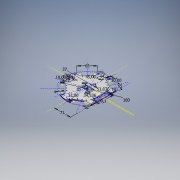
# Autodesk Inventor part: lower_baseplate_collet_alu
Saved by Autodesk Inventor 2018 (Build 220112000, 112)
## iProperties
Created: 2017-08-19
Part Number: lower_baseplate_collet_alu
Material: Aluminum 6061
Document SubType Name: Modeling
Designer: steve
Mass: 141.906 g
Surface Area: 381.464 cm^2
Volume: 52.5578 cm^3
Density: 2.7 g/cm^3
Appearance: Aluminum - Flat
Author: steve
Autodesk Inventor part; units mm, degrees
ref_plane "YZ Plane" through (0, 0, 0) normal (1, 0, 0) x (0, 1, 0)
ref_plane "XZ Plane" through (0, 0, 0) normal (0, 1, 0) x (-1, 0, 0)
ref_plane "XY Plane" through (0, 0, 0) normal (0, 0, 1) x (1, 0, 0)
sketch "Sketch1" plane through (0, 0, 0) normal (0, 0, 1) x (1, 0, 0)
  arc A0 (71, -55.3082) -> (70.1094, -56.433) centre (0, 0) ccw construction
  line L0 (-177.0006, 0) -> (176.9983, 0) construction
  line L1 (0, -176.9989) -> (0, 177.0006) construction
  line L2 (0, 0) -> (-102.7393, 102.7393) construction
  line L3 (0, 0) -> (65.4836, 113.4209) construction
  line L4 (0, 0) -> (-102.7393, -102.7393) construction
  line L5 (0, 0) -> (65.4836, -113.4209) construction
  arc A1 (-63.6396, 63.6396) -> (-82.3264, 36.3644) centre (0, 0) ccw construction
  line L6 (-86.6206, 40.6586) -> (-40.6586, 86.6206) construction
  line L7 (-40.6586, 86.6206) -> (-36.3644, 82.3264) construction
  line L8 (-25.1023, 71.0642) -> (-71.0642, 25.1023)
  line L9 (-71.0642, 25.1023) -> (-82.3264, 36.3644)
  line L10 (-63.6396, 63.6396) -> (-48.0833, 48.0833) construction
  line L11 (5.8542, 75.1397) -> (62.1458, 42.6397)
  line L12 (62.1458, 42.6397) -> (70.1094, 56.433)
  line L13 (73.1458, 61.6923) -> (16.8542, 94.1923) construction
  line L14 (16.8542, 94.1923) -> (13.8177, 88.933) construction
  line L15 (45, 77.9423) -> (34, 58.8897) construction
  line L16 (-36.3644, 82.3264) -> (-25.1023, 71.0642)
  line L17 (-82.3264, 36.3644) -> (-86.6206, 40.6586) construction
  line L18 (13.8177, 88.933) -> (5.8542, 75.1397)
  line L19 (70.1094, 56.433) -> (73.1458, 61.6923) construction
  arc A2 (-36.3644, 82.3264) -> (-63.6396, 63.6396) centre (0, 0) ccw construction
  arc A3 (-82.3264, 36.3644) -> (-90, 0) centre (0, 0) ccw
  arc A4 (13.8177, 88.933) -> (-36.3644, 82.3264) centre (0, 0) ccw
  arc A5 (45, 77.9423) -> (13.8177, 88.933) centre (0, 0) ccw construction
  arc A6 (70.1094, 56.433) -> (45, 77.9423) centre (0, 0) ccw construction
  arc A7 (-90, 0) -> (90, 0) centre (0, 0) ccw construction
  arc A8 (90, 0) -> (71, 55.3082) centre (0, 0) ccw construction
  line L20 (0, 0) -> (-102.7393, -102.7393) construction
  line L21 (0, 0) -> (65.4836, -113.4209) construction
  arc A9 (-82.3264, -36.3644) -> (-63.6396, -63.6396) centre (0, 0) ccw construction
  line L22 (-86.6206, -40.6586) -> (-40.6586, -86.6206) construction
  line L23 (-40.6586, -86.6206) -> (-36.3644, -82.3264) construction
  line L24 (-25.1023, -71.0642) -> (-71.0642, -25.1023)
  line L25 (-71.0642, -25.1023) -> (-82.3264, -36.3644)
  line L26 (-63.6396, -63.6396) -> (-48.0833, -48.0833) construction
  line L27 (5.8542, -75.1397) -> (62.1458, -42.6397)
  line L28 (62.1458, -42.6397) -> (70.1094, -56.433)
  line L29 (73.1458, -61.6923) -> (16.8542, -94.1923) construction
  line L30 (16.8542, -94.1923) -> (13.8177, -88.933) construction
  line L31 (45, -77.9423) -> (34, -58.8897) construction
  line L32 (-36.3644, -82.3264) -> (-25.1023, -71.0642)
  line L33 (-82.3264, -36.3644) -> (-86.6206, -40.6586) construction
  line L34 (13.8177, -88.933) -> (5.8542, -75.1397)
  line L35 (70.1094, -56.433) -> (73.1458, -61.6923) construction
  arc A10 (-63.6396, -63.6396) -> (-36.3644, -82.3264) centre (0, 0) ccw construction
  arc A11 (-90, 0) -> (-82.3264, -36.3644) centre (0, 0) ccw
  arc A12 (-36.3644, -82.3264) -> (13.8177, -88.933) centre (0, 0) ccw
  arc A13 (13.8177, -88.933) -> (45, -77.9423) centre (0, 0) ccw construction
  arc A14 (45, -77.9423) -> (70.1094, -56.433) centre (0, 0) ccw construction
  arc A15 (70.1094, -56.433) -> (71, -55.3082) centre (0, 0) ccw
  line L36 (71, 115.675) -> (71, -111.017) construction
  line L37 (71, -55.3082) -> (71, 55.3082)
  arc A16 (71, 55.3082) -> (70.1094, 56.433) centre (0, 0) ccw
  arc A17 (70.1094, -56.433) -> (71, -55.3082) centre (0, 0) ccw construction
  arc A18 (71, -55.3082) -> (90, 0) centre (0, 0) ccw construction
  dimension "d0" = 180
  dimension "d1" = 45
  dimension "d2" = 30
  dimension "d5" = 22
  dimension "d6" = 65
  dimension "d7" = 22
  dimension "d8" = 65
  dimension "d26" = 71
  constraints: 72 end point, 46 point on circle, 19 centre point, 18 symmetric about line, 9 parallel, 8 perpendicular, 4 midpoint, 4 point on line, 3 coincident, 3 tangent, 2 collinear, 1 vertical, 7 other
  measures "d0" diameter of A0
  measures "d1" angle of L1 L2
  measures "d2" angle of L3 L1
  measures "d5" distance of L6.end L8.start
  measures "d6" distance of L6.start L6.end
  measures "d7" distance of L13.end L11.start
  measures "d8" distance of L13.start L13.end
  measures "d26" distance between parallel lines of L1 L36
extrude "Extrusion1" add sketch "Sketch1" along normal blind 3
sketch "Sketch3" plane through (0, 0, 0) normal (0, 0, -1) x (-1, 0, 0)
  line L0 (0, 0) -> (48.0833, 48.0833) construction
  line L1 (25.1023, 71.0642) -> (71.0642, 25.1023) construction
  line L2 (0, 0) -> (-34, 58.8897) construction
  line L3 (-62.1458, 42.6397) -> (-5.8542, 75.1397) construction
  line L4 (68.9101, 27.2565) -> (27.6205, 68.546) construction
  line L5 (-11.9462, 71.6225) -> (-60.3861, 43.6557) construction
  line L6 (63.8841, 25.9184) -> (21.8996, 67.903) construction
  line L7 (-13.3687, 65.6051) -> (-54.2429, 42.0063) construction
  line L8 (122.2004, 0) -> (-103.2027, 0) construction
  point P0 (44.9013, 44.9013)
  point P1 (-31.75, 54.9926)
  point P2 (54.8008, 35.0018)
  point P3 (-19.6256, 61.9926)
  point P4 (35.0018, 54.8008)
  point P5 (-43.8744, 47.9926)
  point P6 (44.9013, -44.9013)
  point P7 (-31.75, -54.9926)
  point P8 (54.8008, -35.0018)
  point P9 (-19.6256, -61.9926)
  point P10 (35.0018, -54.8008)
  point P11 (-43.8744, -47.9926)
  dimension "d13" = 0
  dimension "d14" = 0
  dimension "d15" = 4.5
  dimension "d16" = 4.5
  dimension "d17" = 14
  dimension "d18" = 14
  constraints: 12 end point, 8 symmetric about line, 6 point on line, 2 midpoint, 2 parallel, 2 perpendicular
  measures "d13" distance between parallel lines of L4 L1
  measures "d14" distance between parallel lines of L5 L3
  measures "d15" distance between parallel lines of L6 L4
  measures "d16" distance between parallel lines of L5 L7
  measures "d17" distance of point (54.801, 35.002) point (44.901, 44.901)
  measures "d18" distance of point (-31.75, 54.993) point (-19.626, 61.993)
hole "Hole1" at (-44.9013, 44.9013, 0) at (31.75, 54.9926, 0) at (-54.8008, 35.0018, 0) at (19.6256, 61.9926, 0) at (-35.0018, 54.8008, 0) at (43.8744, 47.9926, 0) at (-54.8008, -35.0018, 0) at (-44.9013, -44.9013, 0) at (-35.0018, -54.8008, 0) at (19.6256, -61.9926, 0) at (31.75, -54.9926, 0) at (43.8744, -47.9926, 0) direction (0, 0, 1) diameter 3 end through all countersink diameter 6 countersink angle 90
sketch "Sketch5" plane through (0, 0, 3) normal (0, 0, 1) x (1, 0, 0)
  circle A0 centre (31.75, -54.9926) radius 1.5 construction
  circle A1 centre (-35.0018, -54.8008) radius 1.5 construction
  circle A2 centre (-54.8008, -35.0018) radius 1.5 construction
  circle A3 centre (-35.0018, 54.8008) radius 1.5 construction
  circle A4 centre (-54.8008, 35.0018) radius 1.5 construction
  circle A5 centre (-44.9013, 44.9013) radius 1.5 construction
  circle A6 centre (31.75, 54.9926) radius 1.5 construction
  circle A7 centre (19.6256, 61.9926) radius 1.5 construction
  circle A8 centre (43.8744, 47.9926) radius 1.5 construction
  circle A9 centre (-44.9013, -44.9013) radius 1.5 construction
  circle A10 centre (19.6256, -61.9926) radius 1.5 construction
  circle A11 centre (43.8744, -47.9926) radius 1.5 construction
  line L0 (-25.1023, 71.0642) -> (-71.0642, 25.1023) construction
  line L1 (-71.0642, 25.1023) -> (-82.3264, 36.3644) construction
  arc A12 (-82.3264, 36.3644) -> (-82.3264, -36.3644) centre (0, 0) ccw construction
  line L2 (-82.3264, -36.3644) -> (-71.0642, -25.1023) construction
  line L3 (-71.0642, -25.1023) -> (-25.1023, -71.0642) construction
  line L4 (-25.1023, -71.0642) -> (-36.3644, -82.3264) construction
  arc A13 (-36.3644, -82.3264) -> (13.8177, -88.933) centre (0, 0) ccw construction
  line L5 (13.8177, -88.933) -> (5.8542, -75.1397) construction
  line L6 (5.8542, -75.1397) -> (62.1458, -42.6397) construction
  line L7 (62.1458, -42.6397) -> (70.1094, -56.433) construction
  arc A14 (70.1094, -56.433) -> (71, -55.3082) centre (0, 0) ccw construction
  line L8 (71, -55.3082) -> (71, 55.3082) construction
  arc A15 (71, 55.3082) -> (70.1094, 56.433) centre (0, 0) ccw construction
  line L9 (70.1094, 56.433) -> (62.1458, 42.6397) construction
  line L10 (62.1458, 42.6397) -> (5.8542, 75.1397) construction
  line L11 (5.8542, 75.1397) -> (13.8177, 88.933) construction
  arc A16 (13.8177, 88.933) -> (-36.3644, 82.3264) centre (0, 0) ccw construction
  line L12 (-36.3644, 82.3264) -> (-25.1023, 71.0642) construction
  line L13 (71, -55.3082) -> (71, 55.3082) construction
  line L14 (71, -46.5) -> (44, -46.5) construction
  line L15 (44, -46.5) -> (44, 46.5) construction
  line L16 (44, 46.5) -> (71, 46.5) construction
  line L17 (71, 46.5) -> (71, -46.5) construction
  line L18 (71, -31.5) -> (54, -31.5)
  line L19 (54, -31.5) -> (54, 31.5)
  line L20 (54, 31.5) -> (71, 31.5)
  line L21 (71, 31.5) -> (71, -31.5)
  line L22 (-122.2004, 0) -> (103.2027, 0) construction
  line L23 (44, 0) -> (71, 0) construction
  line L24 (54, 0) -> (71, 0) construction
  dimension "d27" = 93
  dimension "d28" = 27
  dimension "d30" = 63
  dimension "d57" = 17
  constraints: 20 end point, 4 midpoint, 4 parallel, 3 perpendicular, 2 collinear, 2 horizontal, 2 point on line
  measures "d27" distance between parallel lines of L16 L14
  measures "d28" distance of L15.end L16.end
  measures "d30" distance of L18.end L19.end
  measures "d57" distance of L18.start L18.end
fillet "Fillet1" radius 10 6 edges at (5.8542, -75.1397, 1.5) (-25.1023, -71.0642, 1.5) (-71.0642, -25.1023, 1.5) (-71.0642, 25.1023, 1.5) (-25.1023, 71.0642, 1.5) (5.8542, 75.1397, 1.5)
ref_plane "Work Plane1" through (0, 0, 3) normal (0, -1, 0) x (1, 0, 0)
extrude "Extrusion3" cut sketch "Sketch5" against normal through all
sketch "Sketch7" plane through (0, 0, 0) normal (0, 0, -1) x (-1, 0, 0)
  line L0 (50.681, 5.7797) -> (-5.2133, -50.1146) construction
  line L1 (63.9932, -32.1734) -> (32.1734, -63.9932) construction
  line L2 (15.0888, -45.3733) -> (-48.6749, -8.5593) construction
  line L3 (-14.5144, -70.1397) -> (-62.1458, -42.6397) construction
  line L4 (33.0572, -11.844) -> (27.4004, -17.5009)
  line L5 (27.4004, -17.5009) -> (25.2791, -15.3796)
  line L6 (25.2791, -15.3796) -> (30.9359, -9.7227)
  line L7 (30.9359, -9.7227) -> (33.0572, -11.844)
  line L8 (0, 0) -> (102.7393, -102.7393) construction
  line L9 (11.844, -33.0572) -> (17.5009, -27.4004)
  line L10 (17.5009, -27.4004) -> (15.3796, -25.2791)
  line L11 (15.3796, -25.2791) -> (9.7227, -30.9359)
  line L12 (9.7227, -30.9359) -> (11.844, -33.0572)
  line L13 (-2.8846, -34.9963) -> (-9.8128, -30.9963)
  line L14 (-9.8128, -30.9963) -> (-8.3878, -28.5281)
  line L15 (-8.3878, -28.5281) -> (-1.4596, -32.5281)
  line L16 (-1.4596, -32.5281) -> (-2.8846, -34.9963)
  line L17 (0, 0) -> (-65.4836, -113.4209) construction
  line L18 (-28.8654, -19.9963) -> (-21.9372, -23.9963)
  line L19 (-21.9372, -23.9963) -> (-20.5122, -21.5281)
  line L20 (-20.5122, -21.5281) -> (-27.4404, -17.5281)
  line L21 (-27.4404, -17.5281) -> (-28.8654, -19.9963)
  line L22 (177.0006, 0) -> (-176.9983, 0) construction
  line L23 (33.0572, 11.844) -> (27.4004, 17.5009)
  line L24 (27.4004, 17.5009) -> (25.2791, 15.3796)
  line L25 (25.2791, 15.3796) -> (30.9359, 9.7227)
  line L26 (30.9359, 9.7227) -> (33.0572, 11.844)
  line L27 (9.7227, 30.9359) -> (11.844, 33.0572)
  line L28 (15.3796, 25.2791) -> (9.7227, 30.9359)
  line L29 (17.5009, 27.4004) -> (15.3796, 25.2791)
  line L30 (11.844, 33.0572) -> (17.5009, 27.4004)
  line L31 (-2.8846, 34.9963) -> (-9.8128, 30.9963)
  line L32 (-9.8128, 30.9963) -> (-8.3878, 28.5281)
  line L33 (-8.3878, 28.5281) -> (-1.4596, 32.5281)
  line L34 (-1.4596, 32.5281) -> (-2.8846, 34.9963)
  line L35 (-27.4404, 17.5281) -> (-28.8654, 19.9963)
  line L36 (-20.5122, 21.5281) -> (-27.4404, 17.5281)
  line L37 (-21.9372, 23.9963) -> (-20.5122, 21.5281)
  line L38 (-28.8654, 19.9963) -> (-21.9372, 23.9963)
  point P0 (-55.5466, -46.4498)
  point P1 (-53.4856, -47.6397)
  dimension "d45" = 36.25
  dimension "d46" = 36.25
  dimension "d47" = 3
  dimension "d48" = 8
  dimension "d49" = 15
  dimension "d51" = 8
  dimension "d52" = 2.85
  dimension "d53" = 15
  constraints: 68 end point, 24 symmetric about line, 4 parallel, 4 perpendicular, 4 point on line
  measures "d45" distance between parallel lines of L0 L1
  measures "d46" distance between parallel lines of L2 L3
  measures "d47" distance of L6.end L4.start
  measures "d48" distance of L5.end L6.end
  measures "d49" distance between parallel lines of L8 L7
  measures "d51" distance of L13.start L13.end
  measures "d52" distance of L15.end L13.start
  measures "d53" distance between parallel lines of L17 L16
extrude "Extrusion2" [suppressed]
fillet "Fillet2" radius 2 10 edges at (13.8177, 88.933, 1.5) (70.1094, 56.433, 1.5) (-82.3264, 36.3644, 1.5) (-36.3644, 82.3264, 1.5) (-82.3264, -36.3644, 1.5) (-36.3644, -82.3264, 1.5) (13.8177, -88.933, 1.5) (70.1094, -56.433, 1.5) (71, -55.3082, 1.5) (71, 55.3082, 1.5)
sketch "Sketch9" plane through (0, 0, 0) normal (0, 0, -1) x (-1, 0, 0)
  line L0 (-54, -31.5) -> (-54, 31.5) construction
  line L1 (-54, 0) -> (-20.2293, 0) construction
  line L2 (-54, -10.05) -> (-19.464, -10.05)
  line L3 (-19.464, -10.05) -> (-19.464, 10.05)
  line L4 (-19.464, 10.05) -> (-54, 10.05)
  line L5 (-54, 10.05) -> (-54, -10.05)
  line L6 (-54, 0) -> (-19.464, 0) construction
  line L7 (-54, 31.5) -> (-54, -31.5) construction
  point P0 (0, 0)
  dimension "d70" = 20.1
  dimension "d71" = 34.536
  constraints: 12 end point, 3 midpoint, 2 collinear, 2 horizontal, 2 parallel, 1 perpendicular
  measures "d70" distance between parallel lines of L2 L4
  measures "d71" distance between parallel lines of L3 L0
sketch "Sketch10" plane through (0, 0, 0) normal (0, 0, -1) x (-1, 0, 0)
  circle A0 centre (0, 0) radius 26 construction
  line L0 (-5.4644, -42.234) -> (43.0476, 6.278) construction
  line L1 (63.9932, -32.1734) -> (32.1734, -63.9932) construction
  line L2 (0, 0) -> (102.7393, -102.7393) construction
  line L3 (20.5061, -20.5061) -> (9.8995, -31.1127) construction
  line L4 (-27.0128, -14.4264) -> (-1.5766, -29.112) construction
  line L5 (-14.5144, -70.1397) -> (-62.1458, -42.6397) construction
  line L6 (-14.5, -25.1147) -> (-27.4904, -17.6147) construction
  line L7 (0, 0) -> (-65.4836, -113.4209) construction
  line L8 (177.0006, 0) -> (-176.9983, 0) construction
  point P0 (18.3848, -18.3848)
  point P1 (31.1127, -9.8995)
  point P2 (-53.4856, -47.6397)
  point P3 (-13, -22.5167)
  point P4 (-1.5096, -32.6147)
  point P5 (9.8995, 31.1127)
  point P6 (18.3848, 18.3848)
  point P7 (31.1127, 9.8995)
  point P8 (-27.4904, 17.6147)
  point P9 (-13, 22.5167)
  point P10 (-1.5096, 32.6147)
  dimension "d72" = 42
  dimension "d75" = 15
  dimension "d76" = 3
  dimension "d77" = 15
  dimension "d78" = 3
  constraints: 8 end point, 8 symmetric about line, 6 point on line, 3 coincident, 2 parallel, 2 perpendicular, 2 tangent, 1 centre point
  measures "d72" distance between parallel lines of L1 L0
  measures "d75" distance of L3.start L3.end
  measures "d76" distance between parallel lines of L0 L3
  measures "d77" distance of L6.start L6.end
  measures "d78" distance between parallel lines of L4 L6
hole "Hole3" [suppressed]
sketch "Sketch11" plane through (0, 0, 0) normal (0, 0, -1) x (-1, 0, 0)
  circle A0 centre (9.0389, -68.6576) radius 17.75 construction
  arc A1 (-10.8406, -89.3447) -> (33.5954, -83.4946) centre (0, 0) ccw construction
  line L0 (11.7474, -89.23) -> (0, 0) construction
  circle A2 centre (9.0389, -68.6576) radius 11 construction
  line L1 (177.0006, 0) -> (-176.9983, 0) construction
  point P0 (11.3558, -86.2557)
  point P1 (10.4747, -79.5635)
  point P2 (17.7658, -61.9612)
  point P3 (-1.1237, -64.448)
  point P4 (10.4747, 79.5635)
  point P5 (17.7658, 61.9612)
  point P6 (-1.1237, 64.448)
  dimension "d86" = 35.5
  dimension "d88" = 22
  dimension "d87" = 3
  dimension "d91" = 360
  constraints: 3 point on line, 3 symmetric about line, 2 end point, 1 coincident, 1 point on circle, 10 other
  measures "d87" distance of L0.start point (11.356, -86.256)
hole "Hole4" at (-10.4747, -79.5635, 0) at (-17.7658, -61.9612, 0) at (1.1237, -64.448, 0) at (-10.4747, 79.5635, 0) at (1.1237, 64.448, 0) at (-17.7658, 61.9612, 0) direction (0, 0, 1) diameter 3 depth 8 tip angle 118 countersink diameter 6 countersink angle 90
sketch "Sketch12" plane through (0, 0, 0) normal (0, 0, -1) x (-1, 0, 0)
  circle A0 centre (-43.8744, 47.9926) radius 1.5 construction
  arc A1 (-67.2679, 51.5115) -> (-71, 50.5115) centre (-69, 50.5115) ccw construction
  line L0 (-62.1458, 42.6397) -> (-14.5144, 70.1397) construction
  line L1 (-62.1458, 42.6397) -> (-14.5144, 70.1397) construction
  line L2 (-45.0474, 52.5115) -> (-69, 52.5115)
  line L3 (-71, 31.5) -> (-54, 31.5) construction
  arc A2 (-67.2679, 51.5115) -> (-71, 50.5115) centre (-69, 50.5115) ccw projected
  arc A3 (-67.2679, 51.5115) -> (-69, 52.5115) centre (-69, 50.5115) ccw construction
  line L4 (-67.2679, 51.5115) -> (-62.1458, 42.6397) construction
  line L5 (-67.2679, 51.5115) -> (-62.1458, 42.6397)
  line L6 (-62.1458, 42.6397) -> (-45.0474, 52.5115) construction
  line L7 (177.0006, 0) -> (-176.9983, 0) construction
  line L8 (-45.0474, 52.5115) -> (-62.1458, 42.6397)
  arc A4 (-67.2679, 51.5115) -> (-69, 52.5115) centre (-69, 50.5115) ccw
  line L9 (-45.0474, -52.5115) -> (-69, -52.5115)
  line L10 (-67.2679, -51.5115) -> (-62.1458, -42.6397)
  line L11 (-45.0474, -52.5115) -> (-62.1458, -42.6397)
  arc A5 (-69, -52.5115) -> (-67.2679, -51.5115) centre (-69, -50.5115) ccw
  point P0 (0, 0)
  constraints: 14 end point, 7 point on circle, 5 symmetric about line, 3 centre point, 2 coincident, 2 collinear, 1 parallel, 1 point on line, 1 tangent, 1 other
extrude "Extrusion5" add sketch "Sketch12" against normal blind 3
fillet "Fillet4" radius 2 2 edges at (45.0474, 52.5115, 1.5) (45.0474, -52.5115, 1.5)
sketch "Sketch13" plane through (0, 0, 3) normal (0, 0, 1) x (1, 0, 0)
  circle A0 centre (0, 0) radius 86 construction
  arc A1 (-63.6396, -63.6396) -> (-36.3644, -82.3264) centre (0, 0) ccw construction
  arc A2 (-90, 0) -> (90, 0) centre (0, 0) ccw construction
  line L0 (0, 0) -> (9.0326, -114.7701) construction
  line L1 (3.7526, -85.9181) -> (9.7341, -85.4473) construction
  line L2 (9.7341, -85.4473) -> (9.2634, -79.4658) construction
  line L3 (9.2634, -79.4658) -> (3.2819, -79.9366) construction
  line L4 (3.2819, -79.9366) -> (3.7526, -85.9181) construction
  line L5 (6.7434, -85.6827) -> (6.2726, -79.7012) construction
  circle A3 centre (-10.4747, -79.5635) radius 1.5 construction
  line L6 (0, 0) -> (-10.4747, -79.5635) construction
  line L7 (3.5172, -82.9273) -> (9.4988, -82.4566) construction
  line L8 (0, 0) -> (-38.4295, -108.5216) construction
  line L9 (-25.862, -82.0192) -> (-31.5178, -80.0164) construction
  line L10 (-31.5178, -80.0164) -> (-29.515, -74.3606) construction
  line L11 (-29.515, -74.3606) -> (-23.8592, -76.3634) construction
  line L12 (-23.8592, -76.3634) -> (-25.862, -82.0192) construction
  line L13 (-28.6899, -81.0178) -> (-26.6871, -75.362) construction
  line L14 (-24.8606, -79.1913) -> (-30.5164, -77.1885) construction
  line L15 (-149.6823, 0) -> (129.9471, 0) construction
  line L16 (0, 0) -> (9.0326, 114.7701) construction
  line L17 (3.7526, 85.9181) -> (9.7341, 85.4473) construction
  line L18 (9.7341, 85.4473) -> (9.2634, 79.4658) construction
  line L19 (9.2634, 79.4658) -> (3.2819, 79.9366) construction
  line L20 (3.2819, 79.9366) -> (3.7526, 85.9181) construction
  line L21 (6.7434, 85.6827) -> (6.2726, 79.7012) construction
  line L22 (3.5172, 82.9273) -> (9.4988, 82.4566) construction
  line L23 (-28.6899, 81.0178) -> (-26.6871, 75.362) construction
  line L24 (-24.8606, 79.1913) -> (-30.5164, 77.1885) construction
  line L25 (-25.862, 82.0192) -> (-31.5178, 80.0164) construction
  line L26 (-29.515, 74.3606) -> (-23.8592, 76.3634) construction
  line L27 (-31.5178, 80.0164) -> (-29.515, 74.3606) construction
  line L28 (-23.8592, 76.3634) -> (-25.862, 82.0192) construction
  line L29 (0, 0) -> (-38.4295, 108.5216) construction
  line L30 (-79.9477, 3) -> (-85.9477, 3) construction
  line L31 (-85.9477, 3) -> (-85.9477, -3) construction
  line L32 (-85.9477, -3) -> (-79.9477, -3) construction
  line L33 (-79.9477, -3) -> (-79.9477, 3) construction
  line L34 (-79.9477, 3) -> (-85.9477, -3) construction
  line L35 (-85.9477, 3) -> (-79.9477, -3) construction
  line L36 (0, 0) -> (-109.7353, -35.6551) construction
  line L37 (-75.1077, -27.5584) -> (-80.814, -29.4125) construction
  line L38 (-80.814, -29.4125) -> (-82.6681, -23.7061) construction
  line L39 (-82.6681, -23.7061) -> (-76.9618, -21.852) construction
  line L40 (-76.9618, -21.852) -> (-75.1077, -27.5584) construction
  line L41 (-75.1077, -27.5584) -> (-82.6681, -23.7061) construction
  line L42 (-80.814, -29.4125) -> (-76.9618, -21.852) construction
  line L43 (-75.1077, 27.5584) -> (-80.814, 29.4125) construction
  line L44 (-80.814, 29.4125) -> (-82.6681, 23.7061) construction
  line L45 (-82.6681, 23.7061) -> (-76.9618, 21.852) construction
  line L46 (-76.9618, 21.852) -> (-75.1077, 27.5584) construction
  line L47 (-75.1077, 27.5584) -> (-82.6681, 23.7061) construction
  line L48 (-80.814, 29.4125) -> (-76.9618, 21.852) construction
  line L49 (-63.9477, -3) -> (-57.9477, -3) construction
  line L50 (-57.9477, -3) -> (-57.9477, 3) construction
  line L51 (-57.9477, 3) -> (-63.9477, 3) construction
  line L52 (-63.9477, 3) -> (-63.9477, -3) construction
  line L53 (-63.9477, -3) -> (-57.9477, 3) construction
  line L54 (-57.9477, -3) -> (-63.9477, 3) construction
  line L55 (-69.9477, -13.35) -> (-69.9477, 15.3078) construction
  point P0 (6.508, -82.692)
  point P1 (6.508, -82.692)
  point P2 (-27.6885, -78.1899)
  point P3 (-27.6885, -78.1899)
  point P4 (6.508, 82.692)
  point P5 (6.508, 82.692)
  point P6 (-27.6885, 78.1899)
  point P7 (-82.9477, 0)
  point P8 (-82.9477, 0)
  point P9 (-78.8879, -25.6322)
  point P10 (-78.8879, 25.6322)
  point P11 (-60.9477, 0)
  point P12 (-60.9477, 0)
  point P13 (-69.9477, -7)
  point P14 (-69.9477, 7)
  point P15 (-27.6885, 78.1899)
  dimension "d103" = 4
  dimension "d104" = 6
  dimension "d105" = 6
  dimension "d106" = 12
  dimension "d114" = 6
  dimension "d115" = 6
  dimension "d171" = 18
  dimension "d172" = 6
  dimension "d173" = 6
  dimension "d174" = 6
  dimension "d175" = 22
  dimension "d183" = 7
  dimension "d184" = 13
  constraints: 110 end point, 39 symmetric about line, 15 midpoint, 9 point on line, 7 parallel, 5 perpendicular, 5 point on circle, 2 coincident, 2 horizontal, 1 centre point, 1 collinear, 1 vertical
  measures "d103" radial gap between concentric circles of A1 A0
  measures "d104" distance of L1.start L1.end
  measures "d105" distance of L1.end L2.end
  measures "d106" angle of L0 L6
  measures "d114" distance of L30.end L31.end
  measures "d115" distance of L30.start L30.end
  measures "d171" angle of L36 L15
  measures "d172" distance of L38.end L39.end
  measures "d173" distance of L39.end L37.start
  measures "d174" distance of L50.end L51.end
  measures "d175" distance of point (-60.948, 0) point (-82.948, 0)
  measures "d183" distance from line of L15 point (-69.948, -7)
  measures "d184" distance from line of point (-82.948, 0) L55
sketch "Sketch6" plane through (0, 0, 0) normal (0, 0, -1) x (-1, 0, 0)
  line L0 (17.036, -61.7264) -> (17.036, 53.4678) construction
  line L1 (-19.964, -41.465) -> (-19.964, 48.4593) construction
  line L2 (-71, -55.3082) -> (-71, 55.3082) construction
  line L3 (-19.964, 9.5) -> (17.036, 9.5) construction
  line L4 (17.036, 9.5) -> (17.036, -9.5) construction
  line L5 (17.036, -9.5) -> (-19.964, -9.5) construction
  line L6 (-19.964, -9.5) -> (-19.964, 9.5) construction
  line L7 (-19.964, 9.5) -> (17.036, -9.5) construction
  line L8 (17.036, 9.5) -> (-19.964, -9.5) construction
  line L9 (-103.6971, 0) -> (122.2828, 0) construction
  line L10 (-51, 34.55) -> (-69, 34.55) construction
  line L11 (-69, 34.55) -> (-69, -34.55) construction
  line L12 (-69, -34.55) -> (-51, -34.55) construction
  line L13 (-51, -34.55) -> (-51, 34.55) construction
  line L14 (-51, 34.55) -> (-69, -34.55) construction
  line L15 (-69, 34.55) -> (-51, -34.55) construction
  line L16 (-71, 31.5) -> (-54, 31.5) construction
  line L17 (-54, 31.5) -> (-54, -31.5) construction
  line L18 (-54, -31.5) -> (-71, -31.5) construction
  line L19 (-71, -50.5115) -> (-71, -31.5) construction
  line L20 (-14.5144, -70.1397) -> (-44.5833, -52.7795) construction
  arc A0 (-10.8542, -83.8) -> (-14.5144, -70.1397) centre (-19.5144, -78.8) ccw construction
  line L21 (-12.3318, -86.3593) -> (-10.8542, -83.8) construction
  arc A1 (-10.8406, -89.3447) -> (33.5954, -83.4946) centre (0, 0) ccw construction
  line L22 (32.1734, -78.1353) -> (34.263, -80.225) construction
  arc A2 (32.1734, -63.9932) -> (32.1734, -78.1353) centre (39.2444, -71.0642) ccw construction
  line L23 (63.9932, -32.1734) -> (32.1734, -63.9932) construction
  arc A3 (78.1353, -32.1734) -> (63.9932, -32.1734) centre (71.0642, -39.2444) ccw construction
  line L24 (80.225, -34.263) -> (78.1353, -32.1734) construction
  arc A4 (83.4946, -33.5954) -> (83.4946, 33.5954) centre (0, 0) ccw construction
  line L25 (78.1353, 32.1734) -> (80.225, 34.263) construction
  arc A5 (63.9932, 32.1734) -> (78.1353, 32.1734) centre (71.0642, 39.2444) ccw construction
  line L26 (32.1734, 63.9932) -> (63.9932, 32.1734) construction
  arc A6 (32.1734, 78.1353) -> (32.1734, 63.9932) centre (39.2444, 71.0642) ccw construction
  line L27 (34.263, 80.225) -> (32.1734, 78.1353) construction
  arc A7 (33.5954, 83.4946) -> (-10.8406, 89.3447) centre (0, 0) ccw construction
  line L28 (-10.8542, 83.8) -> (-12.3318, 86.3593) construction
  arc A8 (-14.5144, 70.1397) -> (-10.8542, 83.8) centre (-19.5144, 78.8) ccw construction
  line L29 (-44.5833, 52.7795) -> (-14.5144, 70.1397) construction
  line L30 (-71, 31.5) -> (-71, 50.5115) construction
  circle A9 centre (-43.8744, -47.9926) radius 3 construction
  circle A10 centre (-19.6256, -61.9926) radius 3 construction
  circle A11 centre (44.9013, -44.9013) radius 3 construction
  circle A12 centre (-43.8744, 47.9926) radius 3 construction
  circle A13 centre (-19.6256, 61.9926) radius 3 construction
  circle A14 centre (-31.75, 54.9926) radius 3 construction
  circle A15 centre (44.9013, 44.9013) radius 3 construction
  circle A16 centre (54.8008, 35.0018) radius 3 construction
  circle A17 centre (35.0018, 54.8008) radius 3 construction
  circle A18 centre (54.8008, -35.0018) radius 3 construction
  circle A19 centre (35.0018, -54.8008) radius 3 construction
  circle A20 centre (-31.75, -54.9926) radius 3 construction
  line L31 (-56, 34.55) -> (-64, 34.55) construction
  line L32 (-64, 34.55) -> (-64, -34.55) construction
  line L33 (-64, -34.55) -> (-56, -34.55) construction
  line L34 (-56, -34.55) -> (-56, 34.55) construction
  line L35 (-56, 34.55) -> (-64, -34.55) construction
  line L36 (-64, 34.55) -> (-56, -34.55) construction
  arc A21 (-69, 52.5115) -> (-71, 50.5115) centre (-69, 50.5115) ccw projected
  arc A22 (-71, -50.5115) -> (-69, -52.5115) centre (-69, -50.5115) ccw projected
  line L37 (-45.5833, -52.5115) -> (-69, -52.5115) projected
  arc A23 (-44.5833, -52.7795) -> (-45.5833, -52.5115) centre (-45.5833, -54.5115) ccw projected
  arc A24 (-12.3318, -86.3593) -> (-10.8406, -89.3447) centre (-10.5997, -87.3593) ccw projected
  arc A25 (33.5954, -83.4946) -> (34.263, -80.225) centre (32.8488, -81.6392) ccw projected
  arc A26 (80.225, -34.263) -> (83.4946, -33.5954) centre (81.6392, -32.8488) ccw projected
  arc A27 (83.4946, 33.5954) -> (80.225, 34.263) centre (81.6392, 32.8488) ccw projected
  arc A28 (34.263, 80.225) -> (33.5954, 83.4946) centre (32.8488, 81.6392) ccw projected
  arc A29 (-10.8406, 89.3447) -> (-12.3318, 86.3593) centre (-10.5997, 87.3593) ccw projected
  arc A30 (-45.5833, 52.5115) -> (-44.5833, 52.7795) centre (-45.5833, 54.5115) ccw projected
  line L38 (-45.5833, 52.5115) -> (-69, 52.5115) projected
  point P0 (-1.464, 0)
  point P1 (-1.464, 0)
  point P2 (-60, 0)
  dimension "d42" = 69.1
  dimension "d43" = 18
  dimension "d44" = 2
  dimension "d61" = 51.036
  dimension "d63" = 37
  dimension "d64" = 19
  dimension "d122" = 5
  constraints: 40 end point, 8 coincident, 7 midpoint, 6 parallel, 5 point on line, 3 horizontal, 3 perpendicular, 2 vertical
  measures "d42" distance between parallel lines of L12 L10
  measures "d43" distance of L10.start L10.end
  measures "d44" distance between parallel lines of L11 L2
  measures "d61" distance between parallel lines of L2 L1
  measures "d63" distance between parallel lines of L0 L1
  measures "d64" distance between parallel lines of L3 L5
  measures "d122" distance between parallel lines of L32 L11
hole "Hole5" at (6.508, -82.692, 3) at (-27.6885, -78.1899, 3) at (-82.9477, 0, 3) at (6.508, 82.692, 3) at (-27.6885, 78.1899, 3) at (-78.8879, -25.6322, 3) at (-78.8879, 25.6322, 3) direction (0, 0, -1) diameter 3 end through all
sketch "Sketch14" plane through (0, 0, 3) normal (0, 0, 1) x (1, 0, 0)
  line L0 (3.2819, -79.9366) -> (3.7526, -85.9181) construction
  line L1 (9.2634, -79.4658) -> (3.2819, -79.9366) construction
  line L2 (9.7341, -85.4473) -> (9.2634, -79.4658) construction
  line L3 (3.7526, -85.9181) -> (9.7341, -85.4473) construction
  line L4 (12.4387, -85.2345) -> (1.7588, -86.075)
  line L5 (1.7588, -86.075) -> (1.2802, -79.9938)
  line L6 (1.2802, -79.9938) -> (11.9601, -79.1533)
  line L7 (11.9601, -79.1533) -> (12.4387, -85.2345)
  arc A0 (10.8406, -89.3447) -> (12.3318, -86.3593) centre (10.5997, -87.3593) ccw construction
  line L8 (0, 0) -> (-10.4747, -79.5635) construction
  line L9 (-34.0752, -79.1108) -> (-23.9767, -82.6869)
  line L10 (-23.9767, -82.6869) -> (-21.9405, -76.9368)
  line L11 (-21.9405, -76.9368) -> (-32.0389, -73.3607)
  line L12 (-32.0389, -73.3607) -> (-34.0752, -79.1108)
  line L13 (-149.6823, 0) -> (129.9471, 0) construction
  line L14 (12.4387, 85.2345) -> (1.7588, 86.075)
  line L15 (1.7588, 86.075) -> (1.2802, 79.9938)
  line L16 (1.2802, 79.9938) -> (11.9601, 79.1533)
  line L17 (11.9601, 79.1533) -> (12.4387, 85.2345)
  line L18 (-32.0389, 73.3607) -> (-34.0752, 79.1108)
  line L19 (-21.9405, 76.9368) -> (-32.0389, 73.3607)
  line L20 (-23.9767, 82.6869) -> (-21.9405, 76.9368)
  line L21 (-34.0752, 79.1108) -> (-23.9767, 82.6869)
  line L22 (-79.9477, 3) -> (-85.9477, -3) construction
  line L23 (-85.9477, 3) -> (-79.9477, -3) construction
  line L24 (-85.9477, 3) -> (-85.9477, -3) construction
  line L25 (-85.9477, -3) -> (-79.9477, -3) construction
  line L26 (-79.9477, -3) -> (-79.9477, 3) construction
  line L27 (-79.8477, -5) -> (-85.9477, -5)
  line L28 (-85.9477, -5) -> (-85.9477, 5)
  line L29 (-85.9477, 5) -> (-79.8477, 5)
  line L30 (-79.8477, 5) -> (-79.8477, -5)
  line L31 (-79.8477, -5) -> (-85.9477, 5) construction
  line L32 (-85.9477, -5) -> (-79.8477, 5) construction
  point P0 (-82.8977, 0)
  dimension "d116" = 0.1
  dimension "d117" = 2
  dimension "d118" = 0.1
  dimension "d119" = 2
  constraints: 44 end point, 12 symmetric about line, 4 parallel, 3 perpendicular, 2 collinear, 2 midpoint, 1 horizontal, 1 point on line, 1 tangent
  measures "d116" distance between parallel lines of L6 L1
  measures "d117" distance between parallel lines of L0 L5
  measures "d118" distance between parallel lines of L30 L26
  measures "d119" distance between parallel lines of L27 L25
extrude "Extrusion6" [suppressed]
hole "Hole6" at (69, 34.55, 0) at (51, 34.55, 0) at (69, -34.55, 0) at (51, -34.55, 0) direction (0, 0, 1) diameter 3 end through all
hole "Hole8" at (-17.036, 9.5, 0) at (-17.036, -9.5, 0) at (19.964, -9.5, 0) at (19.964, 9.5, 0) at (64, -34.55, 0) at (56, -34.55, 0) at (64, 34.55, 0) at (56, 34.55, 0) direction (0, 0, 1) diameter 3 depth 8 tip angle 118 countersink diameter 6 countersink angle 90
sketch "Sketch8" plane through (0, 0, 0) normal (0, 0, -1) x (-1, 0, 0)
  circle A0 centre (17.036, -9.5) radius 1.5 construction
  circle A1 centre (-19.964, -9.275) radius 1.5 construction
  circle A2 centre (-19.964, 9.5) radius 1.5 construction
  circle A3 centre (16.036, 9.275) radius 1.5 construction
  line L0 (17.036, -9.5) -> (-19.964, -9.5) construction
  line L1 (-19.964, -9.5) -> (-19.964, 9.5) construction
  line L2 (-19.964, 9.5) -> (17.036, 9.5) construction
  line L3 (17.036, 9.5) -> (17.036, -9.5) construction
  line L4 (-1.464, -9.5) -> (-1.464, 9.5) construction
  line L5 (17.036, 0) -> (-19.964, 0) construction
  line L6 (-16.464, 10.25) -> (13.536, 10.25)
  line L7 (13.536, 10.25) -> (13.536, -10.25)
  line L8 (13.536, -10.25) -> (-16.464, -10.25)
  line L9 (-16.464, -10.25) -> (-16.464, 10.25)
  line L10 (-16.464, 10.25) -> (13.536, -10.25) construction
  line L11 (13.536, 10.25) -> (-16.464, -10.25) construction
  circle A4 centre (-19.964, -9.5) radius 1.5 construction
  circle A5 centre (-19.964, 9.5) radius 1.5 construction
  circle A6 centre (17.036, 9.5) radius 1.5 construction
  circle A7 centre (17.036, -9.5) radius 1.5 construction
  point P0 (0, 0)
  point P1 (-1.464, 0)
  dimension "d65" = 20.5
  dimension "d66" = 30
  constraints: 24 end point, 7 midpoint, 4 centre point, 4 parallel, 2 horizontal, 2 perpendicular, 1 coincident
  measures "d65" distance of L8.end L6.start
  measures "d66" distance of L7.end L8.end
extrude "Extrusion7" cut sketch "Sketch8" against normal blind 10
sketch "Sketch16" plane through (0, 0, 3) normal (0, 0, 1) x (1, 0, 0)
  line L0 (71, -31.5) -> (54, -31.5) projected
  line L1 (54, -31.5) -> (54, 31.5) projected
  arc A0 (54, -29.3787) -> (56.1213, -31.5) centre (55.0607, -30.4393) ccw
  line L2 (54, -31.5) -> (56.1213, -29.3787) construction
  line L3 (56.1213, -31.5) -> (54, -31.5)
  line L4 (54, -31.5) -> (54, -29.3787)
  line L5 (-122.2, 0) -> (103.2, 0) construction
  arc A1 (56.1213, 31.5) -> (54, 29.3787) centre (55.0607, 30.4393) ccw
  line L6 (56.1213, 31.5) -> (54, 31.5)
  line L7 (54, 31.5) -> (54, 29.3787)
  point P0 (0, 0)
  dimension "d146" = 1.5
  dimension "d147" = 45
  constraints: 10 end point, 6 point on circle, 3 symmetric about line, 2 centre point, 2 point on line, 1 coincident, 1 collinear, 1 midpoint, 1 perpendicular, 1 other
  measures "d146" radius of A0
  measures "d147" angle of L0 L2
extrude "Extrusion8" cut sketch "Sketch16" against normal through all
fillet "Fillet5" radius 1 2 edges at (71, -31.5, 1.5) (71, 31.5, 1.5)
sketch "Sketch17" plane through (0, 0, 3) normal (0, 0, 1) x (1, 0, 0)
  line L0 (28.0228, 18.462) -> (-1.5592, 35.5412) construction
  line L1 (44.5833, 52.7795) -> (14.5144, 70.1397) construction
  circle A0 centre (43.8744, 47.9926) radius 1.5 construction
  arc A1 (70, 31.5) -> (71, 32.5) centre (70, 32.5) ccw construction
  line L2 (71, 32.5) -> (71, 50.5115) construction
  arc A2 (71, 50.5115) -> (69, 52.5115) centre (69, 50.5115) ccw construction
  line L3 (69, 52.5115) -> (45.5833, 52.5115) construction
  arc A3 (44.5833, 52.7795) -> (45.5833, 52.5115) centre (45.5833, 54.5115) ccw construction
  line L4 (44.5833, 52.7795) -> (14.5144, 70.1397) construction
  arc A4 (10.8542, 83.8) -> (14.5144, 70.1397) centre (19.5144, 78.8) ccw construction
  line L5 (10.8542, 83.8) -> (12.3318, 86.3593) construction
  arc A5 (12.3318, 86.3593) -> (10.8406, 89.3447) centre (10.5997, 87.3593) ccw construction
  arc A6 (10.8406, 89.3447) -> (-33.5954, 83.4946) centre (0, 0) ccw construction
  arc A7 (-33.5954, 83.4946) -> (-34.263, 80.225) centre (-32.8488, 81.6392) ccw construction
  line L6 (-34.263, 80.225) -> (-32.1734, 78.1353) construction
  arc A8 (-32.1734, 63.9932) -> (-32.1734, 78.1353) centre (-39.2444, 71.0642) ccw construction
  line L7 (-32.1734, 63.9932) -> (-63.9932, 32.1734) construction
  arc A9 (-78.1353, 32.1734) -> (-63.9932, 32.1734) centre (-71.0642, 39.2444) ccw construction
  line L8 (-78.1353, 32.1734) -> (-80.225, 34.263) construction
  arc A10 (-80.225, 34.263) -> (-83.4946, 33.5954) centre (-81.6392, 32.8488) ccw construction
  arc A11 (-83.4946, 33.5954) -> (-83.4946, -33.5954) centre (0, 0) ccw construction
  arc A12 (-83.4946, -33.5954) -> (-80.225, -34.263) centre (-81.6392, -32.8488) ccw construction
  line L9 (-80.225, -34.263) -> (-78.1353, -32.1734) construction
  arc A13 (-63.9932, -32.1734) -> (-78.1353, -32.1734) centre (-71.0642, -39.2444) ccw construction
  line L10 (-63.9932, -32.1734) -> (-32.1734, -63.9932) construction
  arc A14 (-32.1734, -78.1353) -> (-32.1734, -63.9932) centre (-39.2444, -71.0642) ccw construction
  line L11 (-32.1734, -78.1353) -> (-34.263, -80.225) construction
  arc A15 (-34.263, -80.225) -> (-33.5954, -83.4946) centre (-32.8488, -81.6392) ccw construction
  arc A16 (-33.5954, -83.4946) -> (10.8406, -89.3447) centre (0, 0) ccw construction
  arc A17 (10.8406, -89.3447) -> (12.3318, -86.3593) centre (10.5997, -87.3593) ccw construction
  line L12 (12.3318, -86.3593) -> (10.8542, -83.8) construction
  arc A18 (14.5144, -70.1397) -> (10.8542, -83.8) centre (19.5144, -78.8) ccw construction
  line L13 (14.5144, -70.1397) -> (44.5833, -52.7795) construction
  arc A19 (45.5833, -52.5115) -> (44.5833, -52.7795) centre (45.5833, -54.5115) ccw construction
  line L14 (45.5833, -52.5115) -> (69, -52.5115) construction
  arc A20 (69, -52.5115) -> (71, -50.5115) centre (69, -50.5115) ccw construction
  line L15 (71, -50.5115) -> (71, -32.5) construction
  arc A21 (71, -32.5) -> (70, -31.5) centre (70, -32.5) ccw construction
  line L16 (70, -31.5) -> (56.1213, -31.5) construction
  arc A22 (54, -29.3787) -> (56.1213, -31.5) centre (55.0607, -30.4393) ccw construction
  line L17 (54, -29.3787) -> (54, 29.3787) construction
  arc A23 (56.1213, 31.5) -> (54, 29.3787) centre (55.0607, 30.4393) ccw construction
  line L18 (56.1213, 31.5) -> (70, 31.5) construction
  line L19 (16.464, 10.25) -> (16.464, -10.25) construction
  line L20 (16.464, -10.25) -> (-13.536, -10.25) construction
  line L21 (-13.536, -10.25) -> (-13.536, 10.25) construction
  line L22 (-13.536, 10.25) -> (16.464, 10.25) construction
  circle A24 centre (64, 34.55) radius 1.5 construction
  circle A25 centre (64, -34.55) radius 1.5 construction
  circle A26 centre (19.964, -9.5) radius 1.5 construction
  circle A27 centre (-17.036, 9.5) radius 1.5 construction
  circle A28 centre (-17.036, -9.5) radius 1.5 construction
  circle A29 centre (19.964, 9.5) radius 1.5 construction
  circle A30 centre (56, -34.55) radius 1.5 construction
  circle A31 centre (56, 34.55) radius 1.5 construction
  circle A32 centre (69, -34.55) radius 1.5 construction
  circle A33 centre (69, 34.55) radius 1.5 construction
  circle A34 centre (51, 34.55) radius 1.5 construction
  circle A35 centre (51, -34.55) radius 1.5 construction
  circle A36 centre (6.508, 82.692) radius 1.5 construction
  circle A37 centre (-27.6885, -78.1899) radius 1.5 construction
  circle A38 centre (6.508, -82.692) radius 1.5 construction
  circle A39 centre (-82.9477, 0) radius 1.5 construction
  circle A40 centre (-27.6885, 78.1899) radius 1.5 construction
  circle A41 centre (1.1237, 64.448) radius 1.5 construction
  circle A42 centre (1.1237, -64.448) radius 1.5 construction
  circle A43 centre (-10.4747, -79.5635) radius 1.5 construction
  circle A44 centre (-17.7658, -61.9612) radius 1.5 construction
  circle A45 centre (-10.4747, 79.5635) radius 1.5 construction
  circle A46 centre (-17.7658, 61.9612) radius 1.5 construction
  circle A47 centre (31.75, -54.9926) radius 1.5 construction
  circle A48 centre (-35.0018, -54.8008) radius 1.5 construction
  circle A49 centre (-54.8008, -35.0018) radius 1.5 construction
  circle A50 centre (-35.0018, 54.8008) radius 1.5 construction
  circle A51 centre (-54.8008, 35.0018) radius 1.5 construction
  circle A52 centre (-44.9013, 44.9013) radius 1.5 construction
  circle A53 centre (31.75, 54.9926) radius 1.5 construction
  circle A54 centre (19.6256, 61.9926) radius 1.5 construction
  circle A55 centre (43.8744, 47.9926) radius 1.5 construction
  circle A56 centre (-44.9013, -44.9013) radius 1.5 construction
  circle A57 centre (19.6256, -61.9926) radius 1.5 construction
  circle A58 centre (43.8744, -47.9926) radius 1.5 construction
  line L23 (15, 25.9808) -> (1.1436, 33.9808)
  line L24 (1.1436, 33.9808) -> (-2.8564, 27.0526)
  line L25 (-2.8564, 27.0526) -> (11, 19.0526)
  line L26 (11, 19.0526) -> (15, 25.9808)
  line L27 (-21.2132, 21.2132) -> (-32.5269, 9.8995)
  line L28 (-15.5563, 15.5563) -> (-21.2132, 21.2132)
  line L29 (-26.8701, 4.2426) -> (-15.5563, 15.5563)
  line L30 (-32.5269, 9.8995) -> (-26.8701, 4.2426)
  line L31 (-122.2828, 0) -> (103.6971, 0) construction
  line L32 (0, 0) -> (65.4836, 113.4209) construction
  line L33 (-63.6396, 63.6396) -> (-48.0833, 48.0833) construction
  line L34 (-4.2426, -26.8701) -> (-15.5563, -15.5563)
  line L35 (-15.5563, -15.5563) -> (-21.2132, -21.2132)
  line L36 (-21.2132, -21.2132) -> (-9.8995, -32.5269)
  line L37 (-9.8995, -32.5269) -> (-4.2426, -26.8701)
  line L38 (11, -19.0526) -> (15, -25.9808)
  line L39 (24.8564, -11.0526) -> (11, -19.0526)
  line L40 (28.8564, -17.9808) -> (24.8564, -11.0526)
  line L41 (15, -25.9808) -> (28.8564, -17.9808)
  dimension "d151" = 33.5
  dimension "d152" = 8
  dimension "d157" = 75
  dimension "d161" = 0
  dimension "d162" = 16
  dimension "d165" = 90
  dimension "d169" = 240
  constraints: 34 end point, 3 parallel, 1 perpendicular, 1 point on line, 27 other
  measures "d151" distance from line of L0 A53.centre
  measures "d152" distance between parallel lines of L25 L0
  measures "d161" distance between parallel lines of L26 L32
  measures "d162" distance between parallel lines of L24 L32
extrude "Extrusion9" cut sketch "Sketch17" against normal through all
hole "Hole9" at (-60.9477, 0, 3) at (-69.9477, -7, 3) at (-69.9477, 7, 3) direction (0, 0, -1) diameter 3 end through all
sketch "Sketch18" plane through (0, 0, 3) normal (0, 0, 1) x (1, 0, 0)
  line L0 (-76.9477, -14.4399) -> (-76.9477, 18.3251) construction
  line L1 (-73.6977, -2) -> (-80.1977, -2)
  line L2 (-80.1977, -2) -> (-80.1977, -14)
  line L3 (-80.1977, -14) -> (-73.6977, -14)
  line L4 (-73.6977, -14) -> (-73.6977, -2)
  line L5 (-73.6977, -2) -> (-80.1977, -14) construction
  line L6 (-80.1977, -2) -> (-73.6977, -14) construction
  line L7 (-65.2837, -7) -> (-79.6033, -7) construction
  line L8 (-76.9477, -8) -> (-83.8992, -8) construction
  line L9 (-69.9477, -13.35) -> (-69.9477, 15.3078) construction
  point P0 (0, 0)
  point P1 (-69.9477, -7)
  dimension "d185" = 12
  dimension "d186" = 6.5
  dimension "d187" = 1
  dimension "d188" = 7
  constraints: 18 end point, 3 horizontal, 2 midpoint, 2 parallel, 2 point on line, 1 perpendicular, 1 vertical
  measures "d185" distance between parallel lines of L1 L3
  measures "d186" distance of L2.end L3.end
  measures "d187" distance between parallel lines of L8 L7
  measures "d188" distance between parallel lines of L0 L9
extrude "Extrusion10" cut sketch "Sketch18" against normal through all
fillet "Fillet6" radius 1.5 4 edges at (-73.6977, -14, 1.5) (-80.1977, -14, 1.5) (-80.1977, -2, 1.5) (-73.6977, -2, 1.5)
mirror "Mirror1" about plane through (0, 0, 3) normal (0, -1, 0) of "Fillet6", "Extrusion10"
equation "\"d46\" = d45"
body "Solid1"
